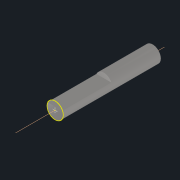
# Autodesk Inventor part: Stepper Motor Axle
Saved by Autodesk Inventor 2021.1 (Build 251245000, 245)
## iProperties
Created: 2020-12-15
Part Number: Stepper Motor Axle
Material: Stainless Steel
Document SubType Name: Modeling
Designer: bestm
Density: 8 g/cm^3
Appearance: Semi-Polished
Author: bestm
Autodesk Inventor part; units mm, degrees
ref_plane "YZ Plane" through (0, 0, 0) normal (1, 0, 0) x (0, 1, 0)
ref_plane "XZ Plane" through (0, 0, 0) normal (0, 1, 0) x (-1, 0, 0)
ref_plane "XY Plane" through (0, 0, 0) normal (0, 0, 1) x (1, 0, 0)
sketch "Sketch1" plane through (0, 0, 0) normal (0, 0, 1) x (1, 0, 0)
  circle A0 centre (0, 0) radius 2.5
  dimension "d0" = 5
  constraints: 1 centre point, 1 coincident
  measures "d0" diameter of A0
extrude "Extrusion1" add sketch "Sketch1" along normal blind 30
sketch "Sketch2" plane through (0, 0, 30) normal (0, 0, 1) x (1, 0, 0)
  line L0 (-2.2913, 1) -> (2.2913, 1)
  circle A0 centre (0, 0) radius 2.5 projected
  dimension "d3" = 1
  constraints: 2 end point, 2 point on circle, 1 horizontal
  measures "d3" distance from line of point (0, 0) L0
extrude "Extrusion2" cut sketch "Sketch2" against normal blind 15 contours A0 L0 picked at (0.534, 1.3064)
body "Solid1"
